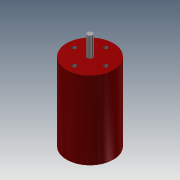
# Autodesk Inventor part: motor-ray
Saved by Autodesk Inventor 2013 (Build 170138000, 138)
## iProperties
Created: 2012-08-14
Part Number: motor-ray
Material: Generic
Document SubType Name: Modeling
Designer: idle-rug
Density: 1 g/cm^3
Author: idle-rug
Autodesk Inventor part; units mm, degrees
ref_plane "YZ Plane" through (0, 0, 0) normal (1, 0, 0) x (0, 1, 0)
ref_plane "XZ Plane" through (0, 0, 0) normal (0, 1, 0) x (-1, 0, 0)
ref_plane "XY Plane" through (0, 0, 0) normal (0, 0, 1) x (1, 0, 0)
sketch "Sketch1" plane through (0, 0, 0) normal (0, 0, 1) x (1, 0, 0)
  circle A0 centre (0, 0) radius 14.1
  dimension "d0" = 28.2
  constraints: 1 centre point, 1 coincident
  measures "d0" diameter of A0
extrude "Extrusion1" add sketch "Sketch1" against normal blind 47
sketch "Sketch2" plane through (0, 0, 0) normal (0, 0, 1) x (1, 0, 0)
  circle A0 centre (0, 0) radius 14.1 projected
  circle A1 centre (0, 0) radius 1.585
  dimension "d3" = 3.17
  constraints: 1 centre point, 1 coincident
  measures "d3" diameter of A1
extrude "Extrusion2" add sketch "Sketch2" along normal blind 12 contours A1
sketch "Sketch3" plane through (0, 0, 0) normal (0, 0, 1) x (1, 0, 0)
  circle A0 centre (-9.5, 0) radius 1.2
  circle A1 centre (9.5, 0) radius 1.2
  circle A2 centre (0, 9.5) radius 1.2
  circle A3 centre (0, -9.5) radius 1.2
  dimension "d8" = 2.4
  dimension "d9" = 2.4
  dimension "d10" = 2.4
  dimension "d11" = 2.4
  constraints: 4 centre point
  measures "d8" diameter of A0
  measures "d9" diameter of A1
  measures "d10" diameter of A2
  measures "d11" diameter of A3
hole "Hole1" at (-9.5, 0, 0) at (0, 9.5, 0) at (9.5, 0, 0) at (0, -9.5, 0) direction (0, 0, -1) diameter 2.459 depth 3 thread size "M3x0.5" designation "M3" class "6H" standard "GB Metric profile"
body "Solid1"
